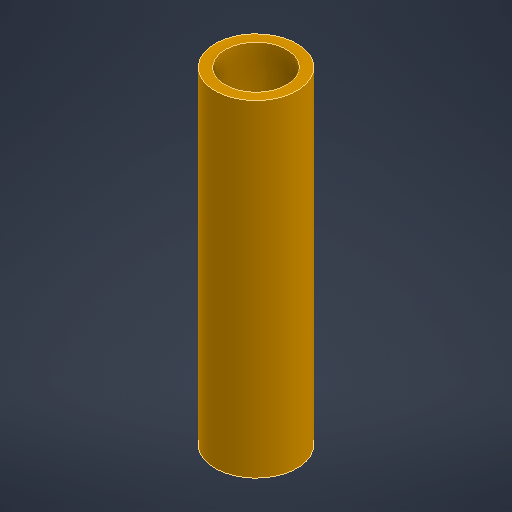
# Autodesk Inventor part: pipe
Saved by Autodesk Inventor 2027 (Build 310192000, 192)
## iProperties
Category: Brass
Company: RoboCrew - Prosek
Created: 2026-03-30
Part Number: pipe
Material: Bronz, měkký cínový
Document SubType Name: Modeling
Designer: Vadim Sobčuk
Density: 8.874 g/cm^3
Appearance: Bronz – satén
Project: MK-1
Checked By: Vadim Sobčuk
Engr Approved By: Vadim Sobčuk
User Status: Manufactured
Mfg Approved By: Vadim Sobčuk
Engineer: Vadim Sobčuk
Authority: Vadim Sobčuk
Author: Vadim Sobčuk
Title: Pipe
Comments: Pro BodyMotor jako kluzný spoj s osou
Autodesk Inventor part; units mm, degrees
ref_plane "YZ Plane" through (0, 0, 0) normal (1, 0, 0) x (0, 1, 0)
ref_plane "XZ Plane" through (0, 0, 0) normal (0, 1, 0) x (-1, 0, 0)
ref_plane "XY Plane" through (0, 0, 0) normal (0, 0, 1) x (1, 0, 0)
sketch "Náčrt1" plane through (0, 0, 0) normal (0, 1, 0) x (-1, 0, 0)
  circle A0 centre (0, 0) radius 2
  circle A1 centre (0, 0) radius 1.5
  dimension "d0" = 4
  dimension "d1" = 3
  constraints: 2 centre point, 2 coincident
  measures "d0" diameter of A0
  measures "d1" diameter of A1
extrude "Vysunutí1" add sketch "Náčrt1" along normal blind 16
